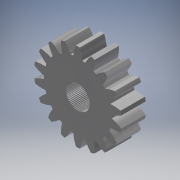
# Autodesk Inventor part: Цилиндрическое зубчатое зацепление1
Saved by Autodesk Inventor 2019 (Build 230136000, 136)
## iProperties
Created: 2020-03-13
Part Number: Цилиндрическое зубчатое зацепление1
Material: Steel
Document SubType Name: Modeling
Designer: Петров Иван
Categories: <?xml version="1.0" encoding="UTF-16"?> <MemberInstance><Categories><FamilyTemplate><FamilyTemplateParameter ValueType="xs:double" Id="1" ObjectReferenceKey="da_z" ObjectType="kUserParameterObject"/><FamilyTemplateParameter ValueType="xs:double" Id="2" ObjectReferenceKey="da_b" ObjectType="kUserParameterObject"/><FamilyTemplateParameter ValueType="xs:double" Id="3" ObjectReferenceKey="da_beta" ObjectType="kUserParameterObject"/><FamilyTemplateParameter ValueType="xs:double" Id="4" ObjectReferenceKey="da_da" ObjectType="kUserParameterObject"/><FamilyTemplateParameter ValueType="xs:double" Id="5" ObjectReferenceKey="da_aw" ObjectType="kUserParameterObject"/><FamilyTemplateParameter ValueType="xs:string" Id="6" ObjectReferenceKey="EAIAABAAAACIAQAAAAAAAIAAAAAAAAAA" ObjectType="83910656" SubObjectId="SurfaceGeometry"/></FamilyTemplate><ParamToTemplateMap><ParamToTemplate CategoryParameter="//CategoryParameter[@InternalName='046C89C9-8512-4d59-83FE-43B91F4F132A']" TemplateParameter="1"/><ParamToTemplate CategoryParameter="//CategoryParameter[@InternalName='2552DF32-E462-4b46-AEBF-C6C7768E72AC']" TemplateParameter="2"/><ParamToTemplate CategoryParameter="//CategoryParameter[@InternalName='C9EE641D-15FC-4fae-A226-E94C4372FDD7']" TemplateParameter="3"/><ParamToTemplate><ParamToTemplate CategoryParameter="//CategoryParameter[@InternalName='00B6519A-459B-49c7-AD84-2E56D39A5744']" ConstantValue="0.000000"/></ParamToTemplate><ParamToTemplate><ParamToTemplate CategoryParameter="//CategoryParameter[@InternalName='04B31F0E-C7A6-4894-AA32-9629BEFACF47']" ConstantValue="1.000000"/></ParamToTemplate><ParamToTemplate><ParamToTemplate CategoryParameter="//CategoryParameter[@InternalName='43CBEC2E-7847-49e7-A936-2F7889FCB2D9']" ConstantValue="0.250000"/></ParamToTemplate><ParamToTemplate><ParamToTemplate CategoryParameter="//CategoryParameter[@InternalName='B1EFC894-105D-4ebd-86BF-FA20ED196853']" ConstantValue="0.350000"/></ParamToTemplate><ParamToTemplate><ParamToTemplate CategoryParameter="//CategoryParameter[@InternalName='51175063-3D10-4879-93E8-6246FE8B403D']" ConstantValue="2060000000.000000"/></ParamToTemplate><ParamToTemplate><ParamToTemplate CategoryParameter="//CategoryParameter[@InternalName='A3A52E27-4454-46a9-B0BD-C932399B70AF']" ConstantValue="0.300000"/></ParamToTemplate><ParamToTemplate><ParamToTemplate CategoryParameter="//CategoryParameter[@InternalName='91B76062-C214-41d9-B1B9-14D2AB99603D']" ConstantValue="0.090000"/></ParamToTemplate><ParamToTemplate><ParamToTemplate CategoryParameter="//CategoryParameter[@InternalName='374E806E-8B8A-4dda-A9AA-1039D6500AD2']" ConstantValue="11.111111"/></ParamToTemplate><ParamToTemplate><ParamToTemplate CategoryParameter="//CategoryParameter[@InternalName='2D373A89-B862-43d6-8D0B-0CBF12AB9F6C']" ConstantValue="0.349066"/></ParamToTemplate><ParamToTemplate CategoryParameter="//CategoryParameter[@InternalName='37777632-D6A2-4fac-9D53-DB8ACD95C989']" TemplateParameter="4"/><ParamToTemplate CategoryParameter="//CategoryParameter[@InternalName='FD1017F1-B727-4f7e-9707-0F86F1FF9423']" TemplateParameter="5"/><ParamToTemplate><ParamToTemplate CategoryParameter="//CategoryParameter[@InternalName='9E1B4470-B2D3-4ff1-B813-535BB4CDF51A']" ConstantValue="3520000.000000"/></ParamToTemplate><ParamToTemplate><ParamToTemplate CategoryParameter="//CategoryParameter[@InternalName='F8452263-BFF6-458c-9FB1-07C4B99E95CD']" ConstantValue="11400000.000000"/></ParamToTemplate><ParamToTemplate><ParamToTemplate CategoryParameter="//CategoryParameter[@InternalName='3E3BB259-FD49-497f-8171-6EBC954A3479']" ConstantValue="2.000000"/></ParamToTemplate><ParamToTemplate CategoryParameter="//CategoryParameter[@InternalName='27C3BAF2-7550-4e4b-AE2C-0DB134B7D9B7']" TemplateParameter="6"/></ParamToTemplateMap><Category DisplayName="Gear" InternalName="DC85795E-93AB-48d5-8EEE-5A27447B64BD" Mnemonic="Gear"><CategoryParameter DisplayName="z" InternalName="046C89C9-8512-4d59-83FE-43B91F4F132A" Mnemonic="z"/><CategoryParameter DisplayName="b" InternalName="2552DF32-E462-4b46-AEBF-C6C7768E72AC" Mnemonic="b"/><CategoryParameter DisplayName="||b|" InternalName="C9EE641D-15FC-4fae-A226-E94C4372FDD7" Mnemonic="beta"/><CategoryParameter DisplayName="x" InternalName="00B6519A-459B-49c7-AD84-2E56D39A5744" Mnemonic="x"/><CategoryParameter DisplayName="a*" InternalName="04B31F0E-C7A6-4894-AA32-9629BEFACF47" Mnemonic="a"/><CategoryParameter DisplayName="c*" InternalName="43CBEC2E-7847-49e7-A936-2F7889FCB2D9" Mnemonic="c"/><CategoryParameter DisplayName="r|.f|*" InternalName="B1EFC894-105D-4ebd-86BF-FA20ED196853" Mnemonic="rf"/><CategoryParameter DisplayName="E" InternalName="51175063-3D10-4879-93E8-6246FE8B403D" Mnemonic="E"/><CategoryParameter DisplayName="||m|" InternalName="A3A52E27-4454-46a9-B0BD-C932399B70AF" Mnemonic="mi"/><Category DisplayName="SpurGear" InternalName="26C5A22E-A91E-4dfd-A3B3-23CCAFAE1764" Mnemonic="SpurGear"><CategoryParameter DisplayName="m" InternalName="91B76062-C214-41d9-B1B9-14D2AB99603D" Mnemonic="m"/><CategoryParameter DisplayName="P" InternalName="374E806E-8B8A-4dda-A9AA-1039D6500AD2" Mnemonic="PP"/><CategoryParameter DisplayName="||a|" InternalName="2D373A89-B862-43d6-8D0B-0CBF12AB9F6C" Mnemonic="alpha"/><CategoryParameter DisplayName="d|.a|" InternalName="37777632-D6A2-4fac-9D53-DB8ACD95C989" Mnemonic="da"/><CategoryParameter DisplayName="a|.w|" InternalName="FD1017F1-B727-4f7e-9707-0F86F1FF9423" Mnemonic="aw"/><CategoryParameter DisplayName="||s||.Flim|" InternalName="9E1B4470-B2D3-4ff1-B813-535BB4CDF51A" Mnemonic="sFlim"/><CategoryParameter DisplayName="||s||.Hlim|" InternalName="F8452263-BFF6-458c-9FB1-07C4B99E95CD" Mnemonic="sHlim"/><CategoryParameter DisplayName="тип" InternalName="3E3BB259-FD49-497f-8171-6EBC954A3479" Mnemonic="type"/><CategoryParameter DisplayName="PitchDiameter" InternalName="27C3BAF2-7550-4e4b-AE2C-0DB134B7D9B7" Mnemonic="IDS_PITCHDIAM"/></Category></Category></Categories></MemberInstance>
Density: 1 g/cm^3
Appearance: Steel
CustomPartVersion: 1
Author: Петров Иван
Autodesk Inventor part; units mm, degrees
sketch "Sketch1" plane through (0, 0, 0) normal (0, 0, 1) x (1, 0, 0)
  circle A0 centre (0, 0) radius 8.9976
  dimension "d0" = 17.9952
  constraints: 1 centre point
  measures "d0" diameter of A0
extrude "Extrusion1" add sketch "Sketch1" along normal blind 5
ref_plane "Work Plane2" through (0, 0, 2.5) normal (0, 0, 1) x (1, 0, 0)
sketch "Sketch2" plane through (0, 0, 0) normal (0, 0, -1) x (-1, 0, 0)
  circle A0 centre (0, 0) radius 8.9976 projected
  circle A1 centre (0, 0) radius 8.05
  dimension "d3" = 16.1
  constraints: 1 centre point, 1 coincident
  measures "d3" diameter of A1
surface extrude "Средний диаметр" sketch "Sketch2" against normal through all shown no curves A1
ref_plane "Work Plane8" through (0, 0, 0) normal (0.9848078, 0.1736482, 0) x (0, 0, 1)
ref_plane "Work Plane9" through (0, 0, 0) normal (1, 0, 0) x (0, 1, 0)
spur gear teeth "Цилиндрическое зубчатое зацепление" teeth 18 pitch diameter 16.2 tip diameter 17.9952 root diameter 13.95 face width 5 start plane through (0, 0, 0) normal (0, 0, -1) x (-1, 0, 0)
sketch "Эскиз3" plane through (0, 0, 5) normal (0, 0, 1) x (1, 0, 0)
  line L0 (0.6049, 2.3742) -> (0.4886, 2.2986)
  line L1 (0.4886, 2.2986) -> (0.4131, 2.4149)
  arc A0 (0.4131, 2.4149) -> (0.3534, 2.4244) centre (0, 0) ccw
  line L2 (0.3534, 2.4244) -> (0.2456, 2.3371)
  line L3 (0.2456, 2.3371) -> (0.1584, 2.4449)
  arc A1 (0.1584, 2.4449) -> (0.098, 2.448) centre (0, 0) ccw
  line L4 (0.098, 2.448) -> (0, 2.35)
  line L5 (0, 2.35) -> (-0.098, 2.448)
  arc A2 (-0.098, 2.448) -> (-0.1584, 2.4449) centre (0, 0) ccw
  line L6 (-0.1584, 2.4449) -> (-0.2456, 2.3371)
  line L7 (-0.2456, 2.3371) -> (-0.3534, 2.4244)
  arc A3 (-0.3534, 2.4244) -> (-0.4131, 2.4149) centre (0, 0) ccw
  line L8 (-0.4131, 2.4149) -> (-0.4886, 2.2986)
  line L9 (-0.4886, 2.2986) -> (-0.6049, 2.3742)
  arc A4 (-0.6049, 2.3742) -> (-0.6632, 2.3585) centre (0, 0) ccw
  line L10 (-0.6632, 2.3585) -> (-0.7262, 2.235)
  line L11 (-0.7262, 2.235) -> (-0.8497, 2.2979)
  arc A5 (-0.8497, 2.2979) -> (-0.9061, 2.2763) centre (0, 0) ccw
  line L12 (-0.9061, 2.2763) -> (-0.9558, 2.1468)
  line L13 (-0.9558, 2.1468) -> (-1.0853, 2.1965)
  arc A6 (-1.0853, 2.1965) -> (-1.1391, 2.1691) centre (0, 0) ccw
  line L14 (-1.1391, 2.1691) -> (-1.175, 2.0352)
  line L15 (-1.175, 2.0352) -> (-1.3089, 2.071)
  arc A7 (-1.3089, 2.071) -> (-1.3596, 2.0381) centre (0, 0) ccw
  line L16 (-1.3596, 2.0381) -> (-1.3813, 1.9012)
  line L17 (-1.3813, 1.9012) -> (-1.5182, 1.9229)
  arc A8 (-1.5182, 1.9229) -> (-1.5652, 1.8848) centre (0, 0) ccw
  line L18 (-1.5652, 1.8848) -> (-1.5725, 1.7464)
  line L19 (-1.5725, 1.7464) -> (-1.7109, 1.7536)
  arc A9 (-1.7109, 1.7536) -> (-1.7536, 1.7109) centre (0, 0) ccw
  line L20 (-1.7536, 1.7109) -> (-1.7464, 1.5725)
  line L21 (-1.7464, 1.5725) -> (-1.8848, 1.5652)
  arc A10 (-1.8848, 1.5652) -> (-1.9229, 1.5182) centre (0, 0) ccw
  line L22 (-1.9229, 1.5182) -> (-1.9012, 1.3813)
  line L23 (-1.9012, 1.3813) -> (-2.0381, 1.3596)
  arc A11 (-2.0381, 1.3596) -> (-2.071, 1.3089) centre (0, 0) ccw
  line L24 (-2.071, 1.3089) -> (-2.0352, 1.175)
  line L25 (-2.0352, 1.175) -> (-2.1691, 1.1391)
  arc A12 (-2.1691, 1.1391) -> (-2.1965, 1.0853) centre (0, 0) ccw
  line L26 (-2.1965, 1.0853) -> (-2.1468, 0.9558)
  line L27 (-2.1468, 0.9558) -> (-2.2763, 0.9061)
  arc A13 (-2.2763, 0.9061) -> (-2.2979, 0.8497) centre (0, 0) ccw
  line L28 (-2.2979, 0.8497) -> (-2.235, 0.7262)
  line L29 (-2.235, 0.7262) -> (-2.3585, 0.6632)
  arc A14 (-2.3585, 0.6632) -> (-2.3742, 0.6049) centre (0, 0) ccw
  line L30 (-2.3742, 0.6049) -> (-2.2986, 0.4886)
  line L31 (-2.2986, 0.4886) -> (-2.4149, 0.4131)
  arc A15 (-2.4149, 0.4131) -> (-2.4244, 0.3534) centre (0, 0) ccw
  line L32 (-2.4244, 0.3534) -> (-2.3371, 0.2456)
  line L33 (-2.3371, 0.2456) -> (-2.4449, 0.1584)
  arc A16 (-2.4449, 0.1584) -> (-2.448, 0.098) centre (0, 0) ccw
  line L34 (-2.448, 0.098) -> (-2.35, 0)
  line L35 (-2.35, 0) -> (-2.448, -0.098)
  arc A17 (-2.448, -0.098) -> (-2.4449, -0.1584) centre (0, 0) ccw
  line L36 (-2.4449, -0.1584) -> (-2.3371, -0.2456)
  line L37 (-2.3371, -0.2456) -> (-2.4244, -0.3534)
  arc A18 (-2.4244, -0.3534) -> (-2.4149, -0.4131) centre (0, 0) ccw
  line L38 (-2.4149, -0.4131) -> (-2.2986, -0.4886)
  line L39 (-2.2986, -0.4886) -> (-2.3742, -0.6049)
  arc A19 (-2.3742, -0.6049) -> (-2.3585, -0.6632) centre (0, 0) ccw
  line L40 (-2.3585, -0.6632) -> (-2.235, -0.7262)
  line L41 (-2.235, -0.7262) -> (-2.2979, -0.8497)
  arc A20 (-2.2979, -0.8497) -> (-2.2763, -0.9061) centre (0, 0) ccw
  line L42 (-2.2763, -0.9061) -> (-2.1468, -0.9558)
  line L43 (-2.1468, -0.9558) -> (-2.1965, -1.0853)
  arc A21 (-2.1965, -1.0853) -> (-2.1691, -1.1391) centre (0, 0) ccw
  line L44 (-2.1691, -1.1391) -> (-2.0352, -1.175)
  line L45 (-2.0352, -1.175) -> (-2.071, -1.3089)
  arc A22 (-2.071, -1.3089) -> (-2.0381, -1.3596) centre (0, 0) ccw
  line L46 (-2.0381, -1.3596) -> (-1.9012, -1.3813)
  line L47 (-1.9012, -1.3813) -> (-1.9229, -1.5182)
  arc A23 (-1.9229, -1.5182) -> (-1.8848, -1.5652) centre (0, 0) ccw
  line L48 (-1.8848, -1.5652) -> (-1.7464, -1.5725)
  line L49 (-1.7464, -1.5725) -> (-1.7536, -1.7109)
  arc A24 (-1.7536, -1.7109) -> (-1.7109, -1.7536) centre (0, 0) ccw
  line L50 (-1.7109, -1.7536) -> (-1.5725, -1.7464)
  line L51 (-1.5725, -1.7464) -> (-1.5652, -1.8848)
  arc A25 (-1.5652, -1.8848) -> (-1.5182, -1.9229) centre (0, 0) ccw
  line L52 (-1.5182, -1.9229) -> (-1.3813, -1.9012)
  line L53 (-1.3813, -1.9012) -> (-1.3596, -2.0381)
  arc A26 (-1.3596, -2.0381) -> (-1.3089, -2.071) centre (0, 0) ccw
  line L54 (-1.3089, -2.071) -> (-1.175, -2.0352)
  line L55 (-1.175, -2.0352) -> (-1.1391, -2.1691)
  arc A27 (-1.1391, -2.1691) -> (-1.0853, -2.1965) centre (0, 0) ccw
  line L56 (-1.0853, -2.1965) -> (-0.9558, -2.1468)
  line L57 (-0.9558, -2.1468) -> (-0.9061, -2.2763)
  arc A28 (-0.9061, -2.2763) -> (-0.8497, -2.2979) centre (0, 0) ccw
  line L58 (-0.8497, -2.2979) -> (-0.7262, -2.235)
  line L59 (-0.7262, -2.235) -> (-0.6632, -2.3585)
  arc A29 (-0.6632, -2.3585) -> (-0.6049, -2.3742) centre (0, 0) ccw
  line L60 (-0.6049, -2.3742) -> (-0.4886, -2.2986)
  line L61 (-0.4886, -2.2986) -> (-0.4131, -2.4149)
  arc A30 (-0.4131, -2.4149) -> (-0.3534, -2.4244) centre (0, 0) ccw
  line L62 (-0.3534, -2.4244) -> (-0.2456, -2.3371)
  line L63 (-0.2456, -2.3371) -> (-0.1584, -2.4449)
  arc A31 (-0.1584, -2.4449) -> (-0.098, -2.448) centre (0, 0) ccw
  line L64 (-0.098, -2.448) -> (0, -2.35)
  line L65 (0, -2.35) -> (0.098, -2.448)
  arc A32 (0.098, -2.448) -> (0.1584, -2.4449) centre (0, 0) ccw
  line L66 (0.1584, -2.4449) -> (0.2456, -2.3371)
  line L67 (0.2456, -2.3371) -> (0.3534, -2.4244)
  arc A33 (0.3534, -2.4244) -> (0.4131, -2.4149) centre (0, 0) ccw
  line L68 (0.4131, -2.4149) -> (0.4886, -2.2986)
  line L69 (0.4886, -2.2986) -> (0.6049, -2.3742)
  arc A34 (0.6049, -2.3742) -> (0.6632, -2.3585) centre (0, 0) ccw
  line L70 (0.6632, -2.3585) -> (0.7262, -2.235)
  line L71 (0.7262, -2.235) -> (0.8497, -2.2979)
  arc A35 (0.8497, -2.2979) -> (0.9061, -2.2763) centre (0, 0) ccw
  line L72 (0.9061, -2.2763) -> (0.9558, -2.1468)
  line L73 (0.9558, -2.1468) -> (1.0853, -2.1965)
  arc A36 (1.0853, -2.1965) -> (1.1391, -2.1691) centre (0, 0) ccw
  line L74 (1.1391, -2.1691) -> (1.175, -2.0352)
  line L75 (1.175, -2.0352) -> (1.3089, -2.071)
  arc A37 (1.3089, -2.071) -> (1.3596, -2.0381) centre (0, 0) ccw
  line L76 (1.3596, -2.0381) -> (1.3813, -1.9012)
  line L77 (1.3813, -1.9012) -> (1.5182, -1.9229)
  arc A38 (1.5182, -1.9229) -> (1.5652, -1.8848) centre (0, 0) ccw
  line L78 (1.5652, -1.8848) -> (1.5725, -1.7464)
  line L79 (1.5725, -1.7464) -> (1.7109, -1.7536)
  arc A39 (1.7109, -1.7536) -> (1.7536, -1.7109) centre (0, 0) ccw
  line L80 (1.7536, -1.7109) -> (1.7464, -1.5725)
  line L81 (1.7464, -1.5725) -> (1.8848, -1.5652)
  arc A40 (1.8848, -1.5652) -> (1.9229, -1.5182) centre (0, 0) ccw
  line L82 (1.9229, -1.5182) -> (1.9012, -1.3813)
  line L83 (1.9012, -1.3813) -> (2.0381, -1.3596)
  arc A41 (2.0381, -1.3596) -> (2.071, -1.3089) centre (0, 0) ccw
  line L84 (2.071, -1.3089) -> (2.0352, -1.175)
  line L85 (2.0352, -1.175) -> (2.1691, -1.1391)
  arc A42 (2.1691, -1.1391) -> (2.1965, -1.0853) centre (0, 0) ccw
  line L86 (2.1965, -1.0853) -> (2.1468, -0.9558)
  line L87 (2.1468, -0.9558) -> (2.2763, -0.9061)
  arc A43 (2.2763, -0.9061) -> (2.2979, -0.8497) centre (0, 0) ccw
  line L88 (2.2979, -0.8497) -> (2.235, -0.7262)
  line L89 (2.235, -0.7262) -> (2.3585, -0.6632)
  arc A44 (2.3585, -0.6632) -> (2.3742, -0.6049) centre (0, 0) ccw
  line L90 (2.3742, -0.6049) -> (2.2986, -0.4886)
  line L91 (2.2986, -0.4886) -> (2.4149, -0.4131)
  arc A45 (2.4149, -0.4131) -> (2.4244, -0.3534) centre (0, 0) ccw
  line L92 (2.4244, -0.3534) -> (2.3371, -0.2456)
  line L93 (2.3371, -0.2456) -> (2.4449, -0.1584)
  arc A46 (2.4449, -0.1584) -> (2.448, -0.098) centre (0, 0) ccw
  line L94 (2.448, -0.098) -> (2.35, 0)
  line L95 (2.35, 0) -> (2.448, 0.098)
  arc A47 (2.448, 0.098) -> (2.4449, 0.1584) centre (0, 0) ccw
  line L96 (2.4449, 0.1584) -> (2.3371, 0.2456)
  line L97 (2.3371, 0.2456) -> (2.4244, 0.3534)
  arc A48 (2.4244, 0.3534) -> (2.4149, 0.4131) centre (0, 0) ccw
  line L98 (2.4149, 0.4131) -> (2.2986, 0.4886)
  line L99 (2.2986, 0.4886) -> (2.3742, 0.6049)
  arc A49 (2.3742, 0.6049) -> (2.3585, 0.6632) centre (0, 0) ccw
  line L100 (2.3585, 0.6632) -> (2.235, 0.7262)
  line L101 (2.235, 0.7262) -> (2.2979, 0.8497)
  arc A50 (2.2979, 0.8497) -> (2.2763, 0.9061) centre (0, 0) ccw
  line L102 (2.2763, 0.9061) -> (2.1468, 0.9558)
  line L103 (2.1468, 0.9558) -> (2.1965, 1.0853)
  arc A51 (2.1965, 1.0853) -> (2.1691, 1.1391) centre (0, 0) ccw
  line L104 (2.1691, 1.1391) -> (2.0352, 1.175)
  line L105 (2.0352, 1.175) -> (2.071, 1.3089)
  arc A52 (2.071, 1.3089) -> (2.0381, 1.3596) centre (0, 0) ccw
  line L106 (2.0381, 1.3596) -> (1.9012, 1.3813)
  line L107 (1.9012, 1.3813) -> (1.9229, 1.5182)
  arc A53 (1.9229, 1.5182) -> (1.8848, 1.5652) centre (0, 0) ccw
  line L108 (1.8848, 1.5652) -> (1.7464, 1.5725)
  line L109 (1.7464, 1.5725) -> (1.7536, 1.7109)
  arc A54 (1.7536, 1.7109) -> (1.7109, 1.7536) centre (0, 0) ccw
  line L110 (1.7109, 1.7536) -> (1.5725, 1.7464)
  line L111 (1.5725, 1.7464) -> (1.5652, 1.8848)
  arc A55 (1.5652, 1.8848) -> (1.5182, 1.9229) centre (0, 0) ccw
  line L112 (1.5182, 1.9229) -> (1.3813, 1.9012)
  line L113 (1.3813, 1.9012) -> (1.3596, 2.0381)
  arc A56 (1.3596, 2.0381) -> (1.3089, 2.071) centre (0, 0) ccw
  line L114 (1.3089, 2.071) -> (1.175, 2.0352)
  line L115 (1.175, 2.0352) -> (1.1391, 2.1691)
  arc A57 (1.1391, 2.1691) -> (1.0853, 2.1965) centre (0, 0) ccw
  line L116 (1.0853, 2.1965) -> (0.9558, 2.1468)
  line L117 (0.9558, 2.1468) -> (0.9061, 2.2763)
  arc A58 (0.9061, 2.2763) -> (0.8497, 2.2979) centre (0, 0) ccw
  line L118 (0.8497, 2.2979) -> (0.7262, 2.235)
  line L119 (0.7262, 2.235) -> (0.6632, 2.3585)
  arc A59 (0.6632, 2.3585) -> (0.6049, 2.3742) centre (0, 0) ccw
  circle A60 centre (0, 0) radius 2.25
  circle A61 centre (0, 0) radius 2.25
  circle A62 centre (0, 0) radius 0.8
  point P0 (5.15, 0)
  constraints: 240 end point, 120 point on circle, 63 centre point
extrude "Выдавливание2" cut sketch "Эскиз3" against normal blind 10 contours A59 L119 L118 A58 L117 L116 A57 L115 L114 A56 L113 L112 A55 L111 L110 A54 L109 L108 A53 L107 L106 A52 L105 L104 A51 L103 L102 A50 L101 L100 A49 L99 L98 A48 L97 L96 A47 L95 L94 A46 L93 L92 A45 L91 L90 A44 L89 L88 A43 L87 L86 A42 L85 L84 A41 L83 L82 A40 L81 L80 A39 L79 L78 A38 L77 L76 A37 L75 L74 A36 L73 L72 A35 L71 L70 A34 L69 L68 A33 L67 L66 A32 L65 L64 A31 L63 L62 A30 L61 L60 A29 L59 L58 A28 L57 L56 A27 L55 L54 A26 L53 L52 A25 L51 L50 A24 L49 L48 A23 L47 L46 A22 L45 L44 A21 L43 L42 A20 L41 L40 A19 L39 L38 A18 L37 L36 A17 L35 L34 A16 L33 L32 A15 L31 L30 A14 L29 L28 A13 L27 L26 A12 L25 L24 A11 L23 L22 A10 L21 L20 A9 L19 L18 A8 L17 L16 A7 L15 L14 A6 L13 L12 A5 L11 L10 A4 L9 L8 A3 L7 L6 A2 L5 L4 A1 L3 L2 A0 L1 L0 | A60 | A62
equation "\"d0\" = da_da"
equation "\"d1\" = da_b"
equation "\"d3\" = da_dw"
equation "\"d46\" = da_aw"
equation "\"d16\" = da_aw"
equation "\"d43\" = da_aw"
equation "\"da_da\" = 17.995235"
equation "\"da_b\" = 5"
equation "\"da_dw\" = 16.1"
equation "\"da_aw\" = 16.1"
body "Solid1"
body "Srf1"
